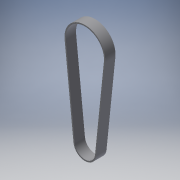
# Autodesk Inventor part: Belt
Saved by Autodesk Inventor 2018 (Build 220112000, 112)
## iProperties
Created: 2017-10-18
Part Number: Belt
Material: Generic
Document SubType Name: Modeling
Designer: Akram Al-Hourani
Density: 1 g/cm^3
Appearance: Default
Author: Akram Al-Hourani
Autodesk Inventor part; units mm, degrees
ref_plane "YZ Plane" through (0, 0, 0) normal (1, 0, 0) x (0, 1, 0)
ref_plane "XZ Plane" through (0, 0, 0) normal (0, 1, 0) x (-1, 0, 0)
ref_plane "XY Plane" through (0, 0, 0) normal (0, 0, 1) x (1, 0, 0)
sketch "Sketch1" plane through (0, 0, 0) normal (0, 1, 0) x (-1, 0, 0)
  arc A0 (-7.9569, -0.8296) -> (7.9569, -0.8296) centre (0, 0) ccw
  line L0 (0, 0) -> (0, 67.5) construction
  arc A1 (14.9191, 65.9444) -> (-14.9191, 65.9444) centre (0, 67.5) ccw
  line L1 (14.9191, 65.9444) -> (7.9569, -0.8296)
  line L2 (-14.9191, 65.9444) -> (-7.9569, -0.8296)
  line L3 (8.9515, -0.9333) -> (15.9137, 65.8407)
  arc A2 (15.9137, 65.8407) -> (-15.9137, 65.8407) centre (0, 67.5) ccw
  line L4 (-15.9137, 65.8407) -> (-8.9515, -0.9333)
  arc A3 (-8.9515, -0.9333) -> (8.9515, -0.9333) centre (0, 0) ccw
  dimension "d0" = 16
  dimension "d1" = 67.5
  dimension "d2" = 30
  dimension "d3" = 1
  constraints: 10 end point, 8 point on circle, 4 centre point, 4 tangent, 2 coincident, 1 vertical, 3 other
  measures "d0" diameter of A0
  measures "d1" distance of L0.start L0.end
  measures "d2" diameter of A1
  measures "d3" distance between parallel lines of L1 L3
extrude "Extrusion1" add sketch "Sketch1" along normal blind 8
body "Solid1"
